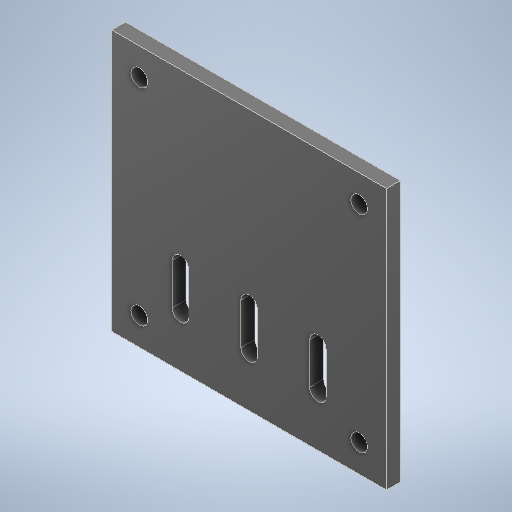
# Autodesk Inventor part: Magazine_Mount_Plate
Saved by Autodesk Inventor 2025.1 (Build 291241020, 241B)
## iProperties
Created: 2024-11-13
Part Number: Magazine_Mount_Plate
Material: PC/ABS Plastic
Document SubType Name: Modeling
Designer: leon-
Density: 1.1 g/cm^3
Appearance: Smooth - Black
Author: leon-
## iProperties of the stored document Magazine_Mount_Plate_3DPrint.ipt
Created: 2024-11-17
Part Number: Magazine_Mount_Plate_3DPrint
Material: Generic
Document SubType Name: Modeling
Designer: leon-
Density: 1 g/cm^3
Appearance: Default
Author: leon-
Autodesk Inventor part; units mm, degrees
ref_plane "YZ Plane" through (0, 0, 0) normal (1, 0, 0) x (0, 1, 0)
ref_plane "XZ Plane" through (0, 0, 0) normal (0, 1, 0) x (-1, 0, 0)
ref_plane "XY Plane" through (0, 0, 0) normal (0, 0, 1) x (1, 0, 0)
sketch "Sketch1" plane through (0, 0, 0) normal (0, 0, 1) x (1, 0, 0)
  line L0 (0, 0) -> (100, 0)
  line L1 (100, 0) -> (100, 95)
  line L2 (100, 95) -> (0, 95)
  line L3 (0, 95) -> (0, 0)
  point P0 (10, 10)
  point P1 (90, 10)
  point P2 (90, 85)
  point P3 (10, 85)
  dimension "d0" = 100
  dimension "d1" = 95
  dimension "d4" = 75
  dimension "d5" = 10
  dimension "d6" = 80
  dimension "d7" = 10
  constraints: 8 end point, 2 horizontal alignment, 2 parallel, 2 vertical alignment, 1 horizontal, 1 perpendicular
  measures "d0" distance of L1.end L2.end
  measures "d1" distance of L0.end L1.end
  measures "d4" distance of point (10, 85) point (10, 10)
  measures "d5" distance from line of L0 point (10, 10)
  measures "d6" distance of point (90, 10) point (10, 10)
  measures "d7" distance from line of L3 point (10, 10)
extrude "Extrusion1" add sketch "Sketch1" along normal blind 5
hole "Hole1" at (10, 10, 0) at (90, 10, 0) at (90, 85, 0) at (10, 85, 0) direction (0, 0, 1) diameter 6 end through all
sketch "Sketch2" plane through (0, 0, 0) normal (0, 0, -1) x (-1, 0, 0)
  line L0 (0, 95) -> (0, 0) projected
  line L1 (-100, 95) -> (0, 95) projected
  line L2 (-75, 33.401) -> (-75, 18.401) construction
  line L3 (-72, 33.401) -> (-72, 18.401)
  line L4 (-78, 18.401) -> (-78, 33.401)
  arc A0 (-72, 33.401) -> (-78, 33.401) centre (-75, 33.401) ccw
  arc A1 (-78, 18.401) -> (-72, 18.401) centre (-75, 18.401) ccw
  line L5 (-50, 33.401) -> (-50, 18.401) construction
  line L6 (-53, 33.401) -> (-53, 18.401)
  line L7 (-47, 18.401) -> (-47, 33.401)
  arc A2 (-47, 33.401) -> (-53, 33.401) centre (-50, 33.401) ccw
  arc A3 (-53, 18.401) -> (-47, 18.401) centre (-50, 18.401) ccw
  line L8 (-25, 33.401) -> (-25, 18.401) construction
  line L9 (-22, 33.401) -> (-22, 18.401)
  line L10 (-28, 18.401) -> (-28, 33.401)
  arc A4 (-22, 33.401) -> (-28, 33.401) centre (-25, 33.401) ccw
  arc A5 (-28, 18.401) -> (-22, 18.401) centre (-25, 18.401) ccw
  point P0 (-25, 25.901)
  point P1 (-50, 25.901)
  point P2 (-75, 25.901)
  point P3 (-75, 25.901)
  point P4 (-50, 25.901)
  point P5 (-25, 25.901)
  dimension "d15" = 50
  dimension "d17" = 25
  dimension "d18" = 25
  dimension "d19" = 69.099
  dimension "d27" = 6
  dimension "d28" = 15
  dimension "d29" = 7.5
  constraints: 24 end point, 12 point on circle, 12 tangent, 6 centre point, 6 horizontal alignment, 6 midpoint, 6 parallel, 2 equal radius, 2 vertical
  measures "d15" distance from line of L0 point (-50, 25.901)
  measures "d17" distance of point (-25, 25.901) point (-50, 25.901)
  measures "d18" distance of point (-50, 25.901) point (-75, 25.901)
  measures "d19" distance from line of L1 point (-50, 25.901)
  measures "d27" distance between parallel lines of L4 L3
  measures "d28" distance of L2.end L2.start
  measures "d29" vertical distance of L3.start point (-75, 25.901)
extrude "Extrusion2" cut sketch "Sketch2" against normal blind 10
equation "\"d29\" = 0.5 * d28"
body "Solid1"
